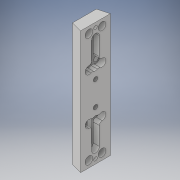
# Autodesk Inventor part: dovetail
Saved by Autodesk Inventor 2019.4 (Build 234330000, 330)
## iProperties
Created: 2020-08-31
Part Number: dovetail
Material: Ogólny
Document SubType Name: Modeling
Designer: barto
Density: 1 g/cm^3
Appearance: Domyślna
Author: barto
Autodesk Inventor part; units mm, degrees
ref_plane "YZ Plane" through (0, 0, 0) normal (1, 0, 0) x (0, 1, 0)
ref_plane "XZ Plane" through (0, 0, 0) normal (0, 1, 0) x (-1, 0, 0)
ref_plane "XY Plane" through (0, 0, 0) normal (0, 0, 1) x (1, 0, 0)
sketch "Szkic1" plane through (0, 0, 0) normal (0, 1, 0) x (-1, 0, 0)
  line L0 (0, 0) -> (0, -43.18)
  line L1 (0, -43.18) -> (15.875, -38.9263)
  line L2 (0, -43.18) -> (16.435, -43.18) construction
  line L3 (0, 0) -> (15.875, -4.2537)
  line L4 (0, 0) -> (18.9194, 0) construction
  line L5 (15.875, -21.59) -> (15.875, -4.2537)
  line L6 (15.875, -21.59) -> (15.875, -38.9263)
  dimension "d0" = 43.18
  dimension "d2" = 15
  dimension "d3" = 15
  dimension "d4" = 15.875
  constraints: 14 end point, 3 vertical, 2 horizontal, 1 equal length
  measures "d0" distance of L0.start L0.end
  measures "d2" angle of L2 L1
  measures "d3" angle of L3 L4
  measures "d4" distance between parallel lines of L0 L6
extrude "Wyciągnięcie proste1" add sketch "Szkic1" along normal blind 177.8
sketch "Szkic2" plane through (0, 0, 0) normal (1, 0, 0) x (0, 0, -1)
  line L0 (0, 0) -> (43.18, 0) projected
  line L1 (0, 177.8) -> (43.18, 177.8) projected
  line L2 (43.18, 0) -> (43.18, 177.8) projected
  line L3 (0, 0) -> (0, 177.8) projected
  point P0 (12.065, 9.525)
  point P1 (12.065, 55.245)
  point P2 (12.065, 122.555)
  point P3 (12.065, 168.275)
  point P4 (31.115, 168.275)
  point P5 (31.115, 122.555)
  point P6 (31.115, 55.245)
  point P7 (31.115, 9.525)
  dimension "d7" = 45.72
  dimension "d8" = 67.31
  dimension "d9" = 45.72
  dimension "d10" = 9.525
  dimension "d12" = 19.05
  dimension "d13" = 19.05
  dimension "d14" = 19.05
  dimension "d15" = 19.05
  dimension "d18" = 12.065
  dimension "d19" = 12.065
  dimension "d20" = 12.065
  dimension "d21" = 12.065
  dimension "d48" = 9.525
  dimension "d49" = 45.72
  dimension "d50" = 67.31
  dimension "d51" = 45.72
  measures "d7" distance of point (12.065, 55.245) point (12.065, 9.525)
  measures "d8" distance of point (12.065, 122.555) point (12.065, 55.245)
  measures "d9" distance of point (12.065, 168.275) point (12.065, 122.555)
  measures "d10" distance from line of L0 point (12.065, 9.525)
  measures "d12" distance of point (12.065, 9.525) point (31.115, 9.525)
  measures "d13" distance of point (12.065, 55.245) point (31.115, 55.245)
  measures "d14" distance of point (12.065, 122.555) point (31.115, 122.555)
  measures "d15" distance of point (12.065, 168.275) point (31.115, 168.275)
  measures "d18" distance from line of L3 point (12.065, 168.275)
  measures "d19" distance from line of L3 point (12.065, 122.555)
  measures "d20" distance from line of L3 point (12.065, 55.245)
  measures "d21" distance from line of L3 point (12.065, 9.525)
  measures "d48" distance from line of L0 point (31.115, 9.525)
  measures "d49" distance of point (31.115, 122.555) point (31.115, 168.275)
  measures "d50" distance of point (31.115, 55.245) point (31.115, 122.555)
  measures "d51" distance of point (31.115, 9.525) point (31.115, 55.245)
hole "Otwór1" at (0, 9.525, -12.065) at (0, 55.245, -12.065) at (0, 122.555, -12.065) at (0, 168.275, -12.065) at (0, 168.275, -31.115) at (0, 122.555, -31.115) at (0, 55.245, -31.115) at (0, 9.525, -31.115) direction (-1, 0, 0) diameter 6.756 depth 30 tip angle 118 counterbore diameter 11.113 counterbore depth 8.89 clearance for "Wkręt z łbem walcowym gniazdowym" size "1/4" standard "ANSI Gwinty cal zunifikowane"
sketch "Szkic3" plane through (-15.875, 0, -38.9263) normal (-1, 0, 0) x (0, 0, 1)
  line L0 (34.6726, 0) -> (34.6726, 177.8) projected
  line L1 (0, 0) -> (0, 177.8) projected
  line L2 (0, 177.8) -> (34.6726, 177.8) projected
  point P0 (38.9263, 0)
  point P1 (17.3366, 106.4)
  point P2 (17.3366, 71.4)
  dimension "d29" = 17.336
  dimension "d31" = 17.336
  dimension "d34" = 35
  dimension "d35" = 71.4
  measures "d29" distance from line of L0 point (17.337, 106.4)
  measures "d31" distance from line of L0 point (17.337, 71.4)
  measures "d34" distance of point (17.337, 106.4) point (17.337, 71.4)
  measures "d35" distance from line of L2 point (17.337, 106.4)
hole "Otwór2" at (-15.875, 106.4, -21.5897) at (-15.875, 71.4, -21.5897) direction (1, 0, 0) diameter 6.401 depth 22.931 tip angle 118 thread size "5/16-18 UNC" class "2B" standard "ANSI Unified Screw Threads"
sketch "Szkic4" plane through (-15.875, 0, -38.9263) normal (-1, 0, 0) x (0, 0, 1)
  line L0 (0, 0) -> (0, 177.8) projected
  line L1 (34.6726, 0) -> (34.6726, 177.8) projected
  circle A0 centre (26.8613, 122.555) radius 5.5565 projected
  circle A1 centre (7.8113, 122.555) radius 3.378 projected
  circle A2 centre (26.8613, 55.245) radius 3.378 projected
  circle A3 centre (7.8113, 55.245) radius 3.378 projected
  arc A4 (13.9583, 122.555) -> (20.7143, 122.555) centre (17.3363, 122.555) ccw
  arc A5 (20.7143, 158.344) -> (13.9583, 158.344) centre (17.3363, 158.344) ccw
  arc A6 (20.7143, 55.245) -> (13.9583, 55.245) centre (17.3363, 55.245) ccw
  arc A7 (13.9583, 19.456) -> (20.7143, 19.456) centre (17.3363, 19.456) ccw
  line L2 (20.7143, 158.344) -> (20.7143, 122.555)
  line L3 (13.9583, 122.555) -> (13.9583, 158.344)
  line L4 (21.3048, 122.555) -> (20.7143, 122.555)
  line L5 (11.1893, 122.555) -> (7.8113, 122.555)
  line L6 (20.7143, 55.245) -> (20.7143, 19.456)
  line L7 (13.9583, 19.456) -> (13.9583, 55.245)
  point P0 (38.9263, 0)
  dimension "d45" = 34.6726
  dimension "d54" = 6.756
  dimension "d55" = 6.756
  dimension "d56" = 6.756
  dimension "d57" = 6.756
  dimension "d66" = 35.789
  dimension "d67" = 35.789
  dimension "d68" = 0
  dimension "d69" = 35.789
  dimension "d70" = 35.789
  constraints: 12 end point, 8 point on circle, 4 centre point, 2 horizontal, 2 horizontal alignment, 2 tangent, 2 other
  measures "d45" distance between parallel lines of L0 L1
  measures "d54" diameter of A4
  measures "d55" diameter of A5
  measures "d56" diameter of A6
  measures "d57" diameter of A7
  measures "d66" distance of L6.start L6.end
  measures "d67" distance of L7.start L7.end
  measures "d68" vertical distance of A2.centre A6.centre
  measures "d69" distance of L2.start L2.end
  measures "d70" distance of L3.start L3.end
extrude "Wyciągnięcie proste2" cut sketch "Szkic4" against normal blind 177.8 contours L3 A5 L2 A4 | L6 A7 L7 A6
sketch "Szkic7" plane through (0, 0, 0) normal (1, 0, 0) x (0, 0, -1)
  arc A0 (18.212, 19.456) -> (24.968, 19.456) centre (21.59, 19.456) ccw projected
  arc A1 (16.0335, 19.456) -> (27.1465, 19.456) centre (21.59, 19.456) ccw
  arc A2 (24.968, 55.245) -> (18.212, 55.245) centre (21.59, 55.245) ccw projected
  arc A3 (27.1465, 55.245) -> (16.0335, 55.245) centre (21.59, 55.245) ccw
  line L0 (16.0335, 19.456) -> (16.0335, 55.245)
  line L1 (27.1465, 19.456) -> (27.1465, 55.245)
  arc A4 (24.968, 158.344) -> (18.212, 158.344) centre (21.59, 158.344) ccw projected
  arc A5 (16.0335, 122.555) -> (27.1465, 122.555) centre (21.59, 122.555) ccw
  arc A6 (27.1465, 158.344) -> (16.0335, 158.344) centre (21.59, 158.344) ccw
  line L2 (16.0335, 122.555) -> (16.0335, 158.344)
  line L3 (27.1465, 122.555) -> (27.1465, 158.344)
  point P0 (0, 0)
  dimension "d71" = 11.113
  dimension "d72" = 11.113
  dimension "d73" = 11.113
  dimension "d74" = 11.113
  constraints: 8 end point, 8 point on circle, 4 centre point, 4 tangent, 3 coincident
  measures "d71" diameter of A1
  measures "d72" diameter of A3
  measures "d73" diameter of A5
  measures "d74" diameter of A6
extrude "Wyciągnięcie proste4" cut sketch "Szkic7" against normal blind 8.89
fillet "Zaokrąglenie1" radius 4 8 edges at (-4.445, 51.3558, -16.0335) (-4.445, 58.1074, -16.8275) (-4.445, 58.1074, -26.3525) (-4.445, 51.3558, -27.1465) (-4.445, 119.6926, -16.8275) (-4.445, 119.6926, -26.3525) (-4.445, 126.4442, -16.0335) (-4.445, 126.4442, -27.1465)
sketch "Szkic8" plane through (-15.875, 0, -38.9263) normal (-1, 0, 0) x (0, 0, 1)
  arc A0 (13.9583, 19.456) -> (20.7143, 19.456) centre (17.3363, 19.456) ccw projected
  line L0 (17.3363, 19.456) -> (17.3363, 202.652)
  line L1 (17.3363, 19.456) -> (17.3363, -13.8574)
  line L2 (0, 177.8) -> (34.6726, 177.8) projected
  line L3 (0, 0) -> (34.6726, 0) projected
  point P0 (38.9263, 0)
  point P1 (17.3363, 6.5)
  point P2 (17.3363, 171.3)
  dimension "d78" = 6.5
  dimension "d79" = 6.5
  constraints: 4 end point, 2 point on line, 2 vertical
  measures "d78" distance from line of L2 point (17.336, 171.3)
  measures "d79" distance from line of L3 point (17.336, 6.5)
hole "Otwór3" at (-15.875, 6.5, -21.59) at (-15.875, 171.3, -21.59) direction (1, 0, 0) diameter 4.978 depth 19.05 tip angle 118 thread size "1/4-20 UNC" class "2B" standard "ANSI Unified Screw Threads"
equation "\"d9\" = d7"
equation "\"d13\" = d12"
equation "\"d14\" = d13"
equation "\"d15\" = d14"
equation "\"d48\" = d10"
equation "\"d49\" = d9"
equation "\"d50\" = d8"
equation "\"d51\" = d7"
equation "\"d31\" = d29"
equation "\"d67\" = d66"
equation "\"d69\" = d66"
equation "\"d70\" = d69"
